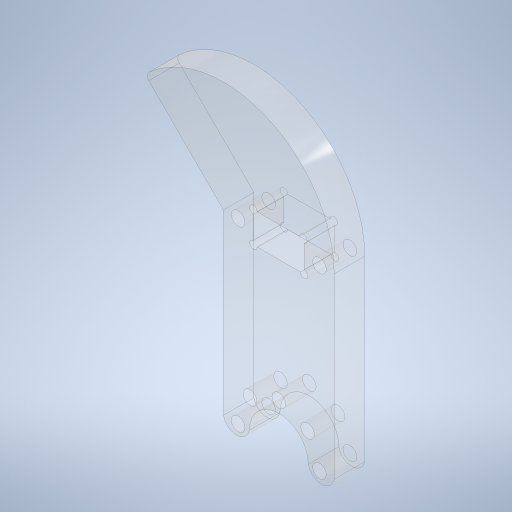
# Autodesk Inventor part: frame_hand1
Saved by Autodesk Inventor 2024 (Build 280153000, 153)
## iProperties
Created: 2024-09-08
Part Number: frame_hand1
Material: PMMA 플라스틱
Document SubType Name: Modeling
Designer: jmha0
Density: 1.188 g/cm^3
Appearance: 폴리카보네이트 - 선명
Mass: 7.6325 g
Surface Area: 33.4737 cm^2
Volume: 6.42466 cm^3
Author: jmha0
Autodesk Inventor part; units mm, degrees
ref_plane "YZ Plane" through (0, 0, 0) normal (1, 0, 0) x (0, 1, 0)
ref_plane "XZ Plane" through (0, 0, 0) normal (0, 1, 0) x (-1, 0, 0)
ref_plane "XY Plane" through (0, 0, 0) normal (0, 0, 1) x (1, 0, 0)
sketch "스케치1" plane through (0, 0, 0) normal (0, 0, 1) x (1, 0, 0)
  circle A0 centre (88.547, 17.9758) radius 1.2
  circle A1 centre (86.2038, 23.6326) radius 1.2
  circle A2 centre (80.547, 25.9758) radius 1.2
  circle A3 centre (74.8901, 23.6326) radius 1.2
  circle A4 centre (72.547, 17.9758) radius 1.2
  circle A5 centre (80.547, 17.9758) radius 5.8
  arc A6 (69.647, 17.9758) -> (74.747, 17.9758) centre (72.197, 18.4832) ccw
  arc A7 (86.347, 17.9758) -> (91.447, 17.9758) centre (88.897, 18.4832) ccw
  line L0 (69.647, 17.9758) -> (91.447, 17.9758)
  line L1 (91.447, 17.9758) -> (91.447, 37.9758)
  line L2 (91.447, 37.9758) -> (69.647, 37.9758)
  line L3 (69.647, 37.9758) -> (69.647, 17.9758)
  line L4 (69.647, 37.9758) -> (99.4042, 37.9758) construction
  line L5 (69.647, 37.9758) -> (91.447, 37.9758)
  line L6 (91.447, 37.9758) -> (91.447, 52.9758)
  line L7 (91.447, 52.9758) -> (69.647, 52.9758)
  line L8 (69.647, 52.9758) -> (69.647, 37.9758)
  line L9 (69.647, 52.9758) -> (69.647, 52.9758)
  line L10 (91.447, 52.9758) -> (91.447, 52.9758)
  circle A8 centre (69.647, 52.9758) radius 21.8
  line L11 (69.647, 52.9758) -> (54.232, 68.3907)
  point P0 (0, 0)
  point P1 (80.547, 17.9758)
  point P2 (80.547, 17.9758)
  point P3 (69.647, 57.9758)
  point P4 (85.4659, 37.9758)
  point P5 (69.647, 31.1758)
  dimension "d4" = 2.6
  dimension "d5" = 2.6
  dimension "d6" = 20
  dimension "d9" = 15
  dimension "d19" = 0
  dimension "d20" = 0
  dimension "d30" = 135
  constraints: 24 end point, 9 centre point, 8 point on circle, 4 parallel, 2 perpendicular, 2 vertical, 1 coincident, 1 collinear, 1 horizontal
  measures "d4" radius of A6
  measures "d5" radius of A7
  measures "d6" distance of L1.end L0.end
  measures "d9" distance of L6.end L1.end
  measures "d19" distance of L7.end L9.end
  measures "d20" distance of L6.end L10.end
  measures "d30" angle of L7 L11
extrude "돌출1" add sketch "스케치1" along normal blind 6 contours L0 A7 A0 | A0 L0 A5 A4 L3 A8 L2 L1 | L2 A8 L6 | A6 L0 A4 | A8 L3 L2 | L2 L8 L7 A8 | L7 L11 A8
sketch "스케치2" plane through (0, 0, 6) normal (0, 0, 1) x (1, 0, 0)
  arc A0 (69.647, 17.9758) -> (74.747, 17.9758) centre (72.197, 18.4832) ccw projected
  arc A1 (86.347, 17.9758) -> (74.747, 17.9758) centre (80.547, 17.9758) ccw projected
  arc A2 (86.347, 17.9758) -> (91.447, 17.9758) centre (88.897, 18.4832) ccw projected
  circle A3 centre (88.547, 17.9758) radius 1.2 projected
  circle A4 centre (72.547, 17.9758) radius 1.2 projected
  circle A5 centre (80.547, 25.9758) radius 1.2 projected
  circle A6 centre (86.2038, 23.6326) radius 1.2 projected
  circle A7 centre (74.8901, 23.6326) radius 1.2 projected
  circle A8 centre (72.547, 17.9758) radius 1.35
  circle A9 centre (74.8901, 23.6326) radius 1.35
  circle A10 centre (80.547, 25.9758) radius 1.35
  circle A11 centre (86.2038, 23.6326) radius 1.35
  circle A12 centre (88.547, 17.9758) radius 1.35
  arc A13 (91.447, 52.9758) -> (54.232, 68.3907) centre (69.647, 52.9758) ccw projected
  line L0 (69.647, 52.9758) -> (69.647, 17.9758) projected
  line L1 (91.447, 17.9758) -> (91.447, 52.9758) projected
  line L2 (54.232, 68.3907) -> (69.647, 52.9758) projected
  point P0 (0, 0)
  dimension "d12" = 2.7
  dimension "d13" = 2.7
  dimension "d14" = 2.7
  dimension "d15" = 2.7
  dimension "d16" = 2.7
  constraints: 5 centre point, 5 coincident
  measures "d12" diameter of A8
  measures "d13" diameter of A9
  measures "d14" diameter of A10
  measures "d15" diameter of A11
  measures "d16" diameter of A12
extrude "돌출2" cut sketch "스케치2" against normal blind 6 contours A3 | A4 | A5 | A6 | A7 | A8 | A9 | A10 | A11 | A12
fillet "모깎기1" radius 1 1 edges at (54.232, 68.3907, 3)
sketch "스케치3" plane through (0, 0, 6) normal (0, 0, 1) x (1, 0, 0)
  arc A0 (54.991, 69.114) -> (54.9562, 67.6666) centre (55.6633, 68.3737) ccw projected
  line L0 (54.9562, 67.6666) -> (69.647, 52.9758) projected
  line L1 (69.647, 52.9758) -> (69.647, 17.9758) projected
  arc A1 (69.647, 17.9758) -> (74.747, 17.9758) centre (72.197, 18.4832) ccw projected
  arc A2 (86.347, 17.9758) -> (74.747, 17.9758) centre (80.547, 17.9758) ccw projected
  arc A3 (86.347, 17.9758) -> (91.447, 17.9758) centre (88.897, 18.4832) ccw projected
  line L2 (91.447, 17.9758) -> (91.447, 52.9758) projected
  arc A4 (91.447, 52.9758) -> (54.991, 69.114) centre (69.647, 52.9758) ccw projected
  circle A5 centre (86.2038, 23.6326) radius 1.35 projected
  circle A6 centre (88.547, 17.9758) radius 1.35 projected
  circle A7 centre (80.547, 25.9758) radius 1.35 projected
  circle A8 centre (72.547, 17.9758) radius 1.35 projected
  circle A9 centre (74.8901, 23.6326) radius 1.35 projected
  line L3 (85.547, 49.9758) -> (75.547, 49.9758)
  line L4 (75.547, 49.9758) -> (75.547, 55.9758)
  line L5 (75.547, 55.9758) -> (85.547, 55.9758)
  line L6 (85.547, 55.9758) -> (85.547, 49.9758)
  line L7 (85.547, 49.9758) -> (75.547, 55.9758) construction
  line L8 (75.547, 49.9758) -> (85.547, 55.9758) construction
  point P0 (0, 0)
  point P1 (80.547, 52.9758)
  dimension "d22" = 10
  dimension "d23" = 6
  constraints: 12 end point, 2 midpoint, 2 parallel, 1 horizontal, 1 perpendicular
  measures "d22" distance of L4.end L5.end
  measures "d23" distance of L3.end L4.end
extrude "돌출3" cut sketch "스케치3" against normal blind 6 contours L3 L4 L5 L6
sketch "스케치4" plane through (0, 0, 6) normal (0, 0, 1) x (1, 0, 0)
  line L0 (75.547, 49.9758) -> (75.547, 55.9758) projected
  line L1 (75.547, 55.9758) -> (85.547, 55.9758) projected
  line L2 (85.547, 55.9758) -> (85.547, 49.9758) projected
  line L3 (85.547, 49.9758) -> (75.547, 49.9758) projected
  arc A0 (54.991, 69.114) -> (54.9562, 67.6666) centre (55.6633, 68.3737) ccw projected
  line L4 (54.9562, 67.6666) -> (69.647, 52.9758) projected
  line L5 (69.647, 52.9758) -> (69.647, 17.9758) projected
  arc A1 (69.647, 17.9758) -> (74.747, 17.9758) centre (72.197, 18.4832) ccw projected
  arc A2 (86.347, 17.9758) -> (74.747, 17.9758) centre (80.547, 17.9758) ccw projected
  arc A3 (86.347, 17.9758) -> (91.447, 17.9758) centre (88.897, 18.4832) ccw projected
  line L6 (91.447, 17.9758) -> (91.447, 52.9758) projected
  arc A4 (91.447, 52.9758) -> (54.991, 69.114) centre (69.647, 52.9758) ccw projected
  circle A5 centre (86.2038, 23.6326) radius 1.35 projected
  circle A6 centre (88.547, 17.9758) radius 1.35 projected
  circle A7 centre (80.547, 25.9758) radius 1.35 projected
  circle A8 centre (72.547, 17.9758) radius 1.35 projected
  circle A9 centre (74.8901, 23.6326) radius 1.35 projected
  circle A10 centre (72.547, 52.9758) radius 1.35
  circle A11 centre (88.547, 52.9758) radius 1.35
  point P0 (0, 0)
  point P1 (75.547, 52.9758)
  dimension "d26" = 2.7
  dimension "d27" = 2.7
  dimension "d31" = 3
  constraints: 2 centre point, 1 midpoint
  measures "d26" diameter of A10
  measures "d27" diameter of A11
  measures "d31" distance of A10.centre point (75.547, 52.976)
extrude "돌출4" cut sketch "스케치4" against normal blind 6 contours A10 | A11
sketch "스케치5" plane through (0, 0, 6) normal (0, 0, 1) x (1, 0, 0)
  line L0 (75.547, 55.9758) -> (75.547, 49.9758) projected
  circle A0 centre (75.547, 55.9758) radius 0.75
  circle A1 centre (85.3736, 55.9758) radius 0.75
  line L1 (75.547, 49.9758) -> (85.547, 49.9758) projected
  circle A2 centre (75.547, 49.9758) radius 0.75
  line L2 (85.547, 49.9758) -> (85.547, 55.9758) projected
  circle A3 centre (85.547, 49.9758) radius 0.75
  point P0 (0, 0)
  point P1 (85.547, 50.7258)
  point P2 (84.797, 49.9758)
  dimension "d32" = 1.5
  dimension "d33" = 1.5
  dimension "d34" = 1.5
  dimension "d35" = 1.5
  constraints: 4 centre point, 2 coincident
  measures "d32" diameter of A0
  measures "d33" diameter of A1
  measures "d34" diameter of A2
  measures "d35" diameter of A3
extrude "돌출5" cut sketch "스케치5" against normal blind 10 contours A1 | L1 L2 A3 | A2 L1 L0 | L0 L1 A2 | A0 picked at (85.0543, 49.916)
